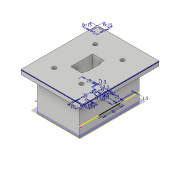
# Autodesk Inventor part: Chamber_coverslip_windowed.v8
Saved by Autodesk Inventor 2017 (Build 210142000, 142)
## iProperties
Created: 2016-07-27
Part Number: Chamber_coverslip_windowed.v8
Material: Generic
Document SubType Name: Modeling
Designer: Craggles
Density: 1 g/cm^3
Appearance: Default
Author: Craggles
Autodesk Inventor part; units mm, degrees
ref_plane "Work Plane1" through (0, 0, 0) normal (0, 0, 1) x (1, 0, 0)
sketch "Sketch1" plane through (0, 0, 0) normal (0, 0, 1) x (1, 0, 0)
  line L0 (45.9471, 19.6712) -> (70.9471, 19.6712)
  line L1 (70.9471, 19.6712) -> (70.9471, 19.8412)
  line L2 (70.9471, 19.8412) -> (45.9471, 19.8412)
  line L3 (45.9471, 19.8412) -> (45.9471, 19.6712)
  line L4 (45.9471, 19.8412) -> (45.9471, 23.669)
  line L5 (45.9471, 23.669) -> (23.5373, 23.669)
  line L6 (24.9679, 22.7263) -> (18.8195, 16.5991) construction
  line L7 (24.9679, 22.7263) -> (19.9679, 22.7263) construction
  line L8 (23.5373, 23.669) -> (24.9679, 22.7263) construction
  line L9 (18.8195, 16.5991) -> (13.8195, 16.5991) construction
  line L10 (13.8195, 16.5991) -> (19.9679, 22.7263)
  line L11 (19.9679, 22.7263) -> (20.9138, 23.669)
  line L12 (20.9138, 23.669) -> (23.5373, 23.669)
  line L13 (63.0355, 15.6366) -> (64.3758, 14.2916) construction
  line L14 (45.9471, 19.6712) -> (43.098, 19.6712) construction
  line L15 (63.0355, 15.6366) -> (65.8803, 15.6366) construction
  line L16 (65.8803, 15.6366) -> (65.8803, 19.8412) construction
  line L17 (72.2599, 24.8293) -> (14.1174, 24.8293)
  line L18 (69.6308, 12.9562) -> (67.6555, 14.9641) construction
  line L19 (69.6308, 12.9562) -> (72.4756, 12.9562) construction
  line L20 (67.6555, 14.9641) -> (70.5003, 14.9641) construction
  line L21 (70.5003, 14.9641) -> (72.4756, 12.9562) construction
  line L22 (70.9471, 14.5099) -> (75.9471, 14.5099) construction
  line L23 (75.9471, 14.5099) -> (75.9471, 24.8293) construction
  line L24 (75.9471, 24.8293) -> (72.2599, 24.8293)
  line L25 (13.8195, 16.5991) -> (11.7231, 14.5099)
  line L26 (11.7231, 14.5099) -> (6.7231, 14.5099) construction
  line L27 (6.7231, 14.5099) -> (6.7231, 24.8293) construction
  line L28 (6.7231, 24.8293) -> (14.1174, 24.8293)
  line L29 (75.9471, 24.8293) -> (6.7231, 24.8293) construction
  line L30 (6.7231, 24.8293) -> (6.7231, 67.9116) construction
  line L31 (6.7231, 67.9116) -> (75.9471, 67.9116)
  line L32 (75.9471, 67.9116) -> (75.9471, 24.8293) construction
  line L33 (11.7231, 14.5099) -> (5.1021, 7.9116)
  line L34 (5.1021, 7.9116) -> (3.1021, 7.9116)
  line L35 (3.1021, 7.9116) -> (3.1021, 67.9116)
  line L36 (3.1021, 67.9116) -> (6.7231, 67.9116)
  line L37 (72.4756, 12.9562) -> (75.9471, 9.4274) construction
  line L38 (5.1021, 7.9116) -> (77.4383, 7.9116) construction
  line L39 (77.4383, 7.9116) -> (75.9471, 9.4274) construction
  line L40 (77.4383, 7.9116) -> (77.4383, 67.9116)
  line L41 (77.4383, 67.9116) -> (75.9471, 67.9116)
  line L42 (77.4383, 7.9116) -> (79.4383, 7.9116)
  line L43 (79.4383, 7.9116) -> (79.4383, 67.9116)
  line L44 (79.4383, 67.9116) -> (77.4383, 67.9116)
  line L45 (70.9471, 19.8412) -> (77.4383, 19.8139)
  line L46 (70.9471, 19.8412) -> (71.4471, 19.8412)
  line L47 (70.9471, 19.8412) -> (71.4471, 19.8412) construction
  line L48 (71.4471, 19.8412) -> (71.4471, 14.0016)
  line L49 (71.4471, 14.0016) -> (77.4383, 7.9116)
  line L50 (45.9471, 19.8412) -> (67.9471, 19.8412)
  line L51 (67.9471, 19.8412) -> (67.9471, 17.5594)
  line L52 (67.9471, 17.5594) -> (71.4471, 14.0016)
  point P0 (0, 0)
  dimension "d0" = 25
  dimension "d1" = 0.17
  dimension "d2" = 5
  dimension "d3" = 5
  dimension "d4" = 2.8492
  dimension "d5" = 2.8448
  dimension "d7" = 2.8448
  dimension "d8" = 2.8448
  dimension "d11" = 5
  dimension "d13" = 5
  dimension "d49" = 2
  dimension "d50" = 2
  dimension "d51" = 90
  dimension "d52" = 0.5
  dimension "d53" = 0
  dimension "d54" = 90
  dimension "d175" = 60
  dimension "d199" = 22
  constraints: 106 end point, 15 horizontal, 8 perpendicular, 8 point on line, 6 parallel, 4 collinear
  measures "d0" distance of L2.end L1.end
  measures "d1" distance of L1.end L0.end
  measures "d2" distance of L6.start L7.end
  measures "d3" distance of L6.end L9.end
  measures "d4" distance of L0.start L14.end
  measures "d5" distance of L13.start L15.end
  measures "d7" distance of L18.start L19.end
  measures "d8" distance of L18.end L20.end
  measures "d11" distance of L22.start L23.start
  measures "d13" distance of L25.end L26.end
  measures "d49" distance of L33.end L34.end
  measures "d50" distance of L38.end L42.end
  measures "d51" angle of L43 L42
  measures "d52" distance of L1.end L46.end
  measures "d53" distance between parallel lines of L46 L47
  measures "d54" angle of L46 L48
  measures "d175" distance between parallel lines of L36 L34
  measures "d199" distance of L2.end L50.end
extrude "Extrusion1" add sketch "Sketch1" along normal mid plane 59.125 contours L51 L2 L1 L0 | L0 L1 L45 L48 L52 L51 | L4 L5 L12 L11 L10 L25 L33 L34 L35 L36 L31 L41 L40 L45 L48 L46 L2 | L46 L48 L45 | L48 L45 L40 L49 | L40 L44 L43 L42
sketch "Sketch3" plane through (0, 0, -29.5625) normal (0, 0, -1) x (-1, 0, 0)
  line L0 (-79.4383, 7.9116) -> (-77.4383, 7.9116) projected
  line L1 (-3.1021, 67.9116) -> (-79.4383, 67.9116)
  line L2 (-79.4383, 67.9116) -> (-79.4383, 7.9116)
  line L3 (-79.4383, 7.9116) -> (-3.1021, 7.9116)
  line L4 (-3.1021, 7.9116) -> (-3.1021, 67.9116)
  point P0 (-3.1021, 7.9116)
  constraints: 8 end point, 2 parallel, 1 horizontal, 1 perpendicular
extrude "End" add sketch "Sketch3" along normal blind 25
sketch "Sketch4" plane through (0, 0, 29.5625) normal (0, 0, 1) x (1, 0, 0)
  line L0 (3.1021, 67.9116) -> (3.1021, 7.9116) projected
  line L1 (79.4383, 7.9116) -> (3.1021, 7.9116)
  line L2 (3.1021, 7.9116) -> (3.1021, 67.9116)
  line L3 (3.1021, 67.9116) -> (79.4383, 67.9116)
  line L4 (79.4383, 67.9116) -> (79.4383, 7.9116)
  constraints: 8 end point, 2 parallel, 1 horizontal, 1 perpendicular
extrude "EndII" add sketch "Sketch4" along normal blind 25
sketch "Sketch7" plane through (45.9471, 19.8412, 29.5625) normal (0, -1, 0) x (1, 0, 0)
  line L0 (0, -18.5625) -> (5, -18.5625)
  line L1 (5, -18.5625) -> (5, -40.5625)
  line L2 (5, -40.5625) -> (0, -40.5625)
  line L3 (0, -40.5625) -> (0, -18.5625)
  line L4 (0, -59.125) -> (0, 0) projected
  point P0 (-45.9471, -29.5625)
  point P1 (0, -29.5625)
  dimension "d24" = 5
  dimension "d25" = 22
  constraints: 8 end point, 2 midpoint, 2 parallel, 1 horizontal, 1 perpendicular
  measures "d24" distance of L1.end L2.end
  measures "d25" distance of L0.end L1.end
extrude "Extrusion4" cut sketch "Sketch7" against normal up to surface (3.8278 mm away)
sketch "Sketch8" plane through (0, 0, 0) normal (0, 0, 1) x (1, 0, 0)
  point P0 (0, 0)
sketch "Sketch9" plane through (45.9471, 19.8412, -29.5625) normal (0, -1, 0) x (1, 0, 0)
  line L0 (25, 59.125) -> (25, 0) projected
  line L1 (0, 40.5625) -> (25, 40.5625)
  line L2 (25, 40.5625) -> (25, 41.5625)
  line L3 (25, 41.5625) -> (0, 41.5625)
  line L4 (0, 41.5625) -> (0, 40.5625)
  line L5 (0, 18.5625) -> (25, 18.5625)
  line L6 (25, 18.5625) -> (25, 17.5625)
  line L7 (25, 17.5625) -> (0, 17.5625)
  line L8 (0, 17.5625) -> (0, 18.5625)
  line L9 (0, 0) -> (0, 18.5625) projected
  line L10 (25, 17.5625) -> (0, 17.5625)
  line L11 (0, 17.5625) -> (0, 18.0625)
  line L12 (0, 18.0625) -> (25, 18.0625)
  line L13 (25, 18.0625) -> (25, 17.5625)
  line L14 (25, 41.5625) -> (0, 41.5625)
  line L15 (0, 41.5625) -> (0, 41.0625)
  line L16 (0, 41.0625) -> (25, 41.0625)
  line L17 (25, 41.0625) -> (25, 41.5625)
  point P0 (-45.9471, 29.5625)
  dimension "d28" = 1
  dimension "d29" = 1
  constraints: 32 end point, 8 parallel, 4 horizontal, 4 perpendicular, 3 point on line, 1 midpoint
  measures "d28" distance of L2.end L1.end
  measures "d29" distance of L5.end L6.end
extrude "Extrusion8" add sketch "Sketch9" along normal blind 0.1 contours L0 L16 L4 L3 | L0 L7 L8 L12
ref_plane "Work Plane2" through (45.9471, 26.669, -11) normal (0, -1, 0) x (1, 0, 0)
sketch "Sketch12" plane through (45.9471, 26.669, -11) normal (0, -1, 0) x (1, 0, 0)
  point P0 (-45.9471, 11)
sketch "Sketch14" plane through (45.9471, 26.669, -11) normal (0, -1, 0) x (1, 0, 0)
  line L0 (-42.845, -43.5625) -> (-42.845, 65.5625) projected
  line L1 (33.4911, -43.5625) -> (33.4911, 65.5625) projected
  line L2 (33.4911, 30) -> (33.4911, -8)
  line L3 (-42.845, -8) -> (-42.845, 30)
  line L4 (-42.845, -43.5625) -> (-42.845, 65.5625) projected
  line L5 (-42.845, 30) -> (-17.845, 30)
  line L6 (-17.845, 30) -> (-17.845, -8)
  line L7 (-17.845, -8) -> (-42.845, -8)
  line L8 (-42.845, -8) -> (-42.845, 30)
  line L9 (33.4911, 30) -> (8.4911, 30)
  line L10 (8.4911, 30) -> (8.4911, -8)
  line L11 (8.4911, -8) -> (33.4911, -8)
  line L12 (33.4911, -8) -> (33.4911, 30)
  line L13 (-17.845, 30) -> (-17.845, -8)
  line L14 (8.4911, -8) -> (8.4911, 30)
  line L15 (-17.845, 30) -> (-15.845, 30)
  line L16 (-15.845, 30) -> (-15.845, -8)
  line L17 (-15.845, -8) -> (-17.845, -8)
  line L18 (-17.845, -8) -> (-17.845, 30)
  line L19 (8.4911, 30) -> (6.4911, 30)
  line L20 (6.4911, 30) -> (6.4911, -8)
  line L21 (6.4911, -8) -> (8.4911, -8)
  line L22 (8.4911, -8) -> (8.4911, 30)
  line L23 (-15.845, -8) -> (-15.845, 30)
  line L24 (6.4911, 30) -> (6.4911, -8)
  line L25 (-15.845, -8) -> (-15.845, 30)
  line L26 (-15.845, 30) -> (-15.845, -8)
  line L27 (0, 22) -> (0, 40.5625) projected
  line L28 (-17.845, -8) -> (0, -8)
  line L29 (0, -8) -> (0, 30)
  line L30 (0, 30) -> (-17.845, 30)
  line L31 (-17.845, 30) -> (-17.845, -8)
  line L32 (5, 22) -> (5, 0) projected
  line L33 (0, 22) -> (5, 22)
  line L34 (5, 22) -> (5, 0)
  line L35 (5, 0) -> (0, 0)
  line L36 (0, 0) -> (0, 22)
  line L37 (1.5, 31.5) -> (-17.345, 31.5)
  line L38 (-17.345, 31.5) -> (-17.345, -9.5)
  line L39 (-17.345, -9.5) -> (1.5, -9.5)
  line L40 (1.5, -9.5) -> (1.5, 31.5)
  line L41 (6.5, 23.5) -> (0, 23.5)
  line L42 (0, 23.5) -> (0, -1.5)
  line L43 (0, -1.5) -> (6.5, -1.5)
  line L44 (6.5, -1.5) -> (6.5, 23.5)
  point P0 (-45.9471, 11)
  point P1 (-45.845, 65.5625)
  point P2 (36.4911, 65.5625)
  point P3 (-42.845, 11)
  point P4 (-42.845, 11)
  dimension "d55" = 38
  dimension "d58" = 25
  dimension "d59" = 38
  dimension "d60" = 25
  dimension "d135" = 2
  dimension "d136" = 2
  dimension "d153" = 1.5
  dimension "d154" = 1.5
  dimension "d155" = 1.5
  dimension "d156" = 1.5
  dimension "d157" = 1.5
  dimension "d158" = 1.5
  dimension "d159" = 1.5
  constraints: 80 end point, 19 parallel, 8 horizontal, 8 perpendicular, 3 point on line, 1 coincident, 1 midpoint, 6 other
  measures "d55" distance of L2.start L2.end
  measures "d58" distance of L6.end L7.end
  measures "d59" distance of L5.end L6.end
  measures "d60" distance of L11.end L10.end
  measures "d135" distance of L16.end L17.end
  measures "d136" distance of L21.end L20.end
  measures "d153" distance between parallel lines of L38 L16
  measures "d154" distance between parallel lines of L39 L28
  measures "d155" distance between parallel lines of L40 L29
  measures "d156" distance between parallel lines of L37 L30
  measures "d157" distance between parallel lines of L33 L41
  measures "d158" distance between parallel lines of L32 L44
  measures "d159" distance between parallel lines of L43 L35
extrude "Extrusion10" cut sketch "Sketch14" against normal blind 5 contours L0 L5 L6 L7
ref_plane "Work Plane3" through (0.1021, 7.9116, 54.5625) normal (0, -1, 0) x (1, 0, 0)
sketch "Sketch17" plane through (3.1021, 67.9116, -54.5625) normal (0, 1, 0) x (1, 0, 0)
  line L0 (82.3362, -109.125) -> (0, -109.125) projected
  line L1 (0, -109.125) -> (76.3362, -109.125)
  line L2 (76.3362, -109.125) -> (76.3362, 0)
  line L3 (76.3362, 0) -> (0, 0)
  line L4 (0, 0) -> (0, -109.125)
  point P0 (-3.1021, -54.5625)
  constraints: 8 end point, 2 parallel, 1 horizontal, 1 perpendicular
extrude "Extrusion11" add sketch "Sketch17" along normal blind 10
ref_plane "Work Plane4" through (3.1021, 77.9116, -54.5625) normal (0, 1, 0) x (1, 0, 0)
sketch "Sketch18" plane through (3.1021, 77.9116, -54.5625) normal (0, 1, 0) x (1, 0, 0)
  line L0 (0, 0) -> (-15, 0) construction
  line L1 (-15, 0) -> (-15, 15)
  line L2 (-15, 15) -> (0, 15)
  line L3 (0, 15) -> (0, 0) construction
  line L4 (82.3362, -109.125) -> (97.3362, -109.125) construction
  line L5 (97.3362, -109.125) -> (97.3362, -124.125)
  line L6 (97.3362, -124.125) -> (82.3362, -124.125)
  line L7 (82.3362, -124.125) -> (82.3362, -109.125) construction
  line L8 (97.3362, -124.125) -> (-15, -124.125)
  line L9 (-15, -124.125) -> (-15, 15)
  line L10 (-15, 15) -> (97.3362, 15)
  line L11 (97.3362, 15) -> (97.3362, -124.125)
  line L12 (-15, 15) -> (-13, 15)
  line L13 (-13, 15) -> (-13, 13)
  line L14 (-13, 13) -> (-15, 13)
  line L15 (-15, 13) -> (-15, 15)
  line L16 (97.3362, -124.125) -> (95.3362, -124.125)
  line L17 (95.3362, -124.125) -> (95.3362, -122.125)
  line L18 (95.3362, -122.125) -> (97.3362, -122.125)
  line L19 (97.3362, -122.125) -> (97.3362, -124.125)
  line L20 (-13, 13) -> (95.3362, 13)
  line L21 (95.3362, 13) -> (95.3362, -122.125)
  line L22 (95.3362, -122.125) -> (-13, -122.125)
  line L23 (-13, -122.125) -> (-13, 13)
  line L24 (-13, 15) -> (-15, 15)
  line L25 (-15, 15) -> (-15, -124.125)
  line L26 (-15, -124.125) -> (-13, -124.125)
  line L27 (-13, -124.125) -> (-13, 15)
  line L28 (97.3362, 15) -> (95.3362, 15)
  line L29 (95.3362, 15) -> (95.3362, -124.125)
  line L30 (95.3362, -124.125) -> (97.3362, -124.125)
  line L31 (97.3362, -124.125) -> (97.3362, 15)
  point P0 (-3.1021, -54.5625)
  point P1 (0, 0)
  dimension "d106" = 15
  dimension "d107" = 15
  dimension "d108" = 15
  dimension "d109" = 15
  dimension "d110" = 2
  dimension "d111" = 2
  dimension "d112" = 2
  dimension "d113" = 2
  constraints: 64 end point, 16 parallel, 8 horizontal, 8 perpendicular, 1 coincident
  measures "d106" distance of L1.end L2.end
  measures "d107" distance of L0.end L1.end
  measures "d108" distance of L5.end L6.end
  measures "d109" distance of L4.end L5.end
  measures "d110" distance of L13.end L14.end
  measures "d111" distance of L12.end L13.end
  measures "d112" distance of L17.end L18.end
  measures "d113" distance of L16.end L17.end
extrude "Extrusion15" add sketch "Sketch18" along normal blind 1
extrude "Extrusion16" add sketch "Sketch18" against normal blind 7.5 contours L1 L14 L23 L27 L8 L9 | L1 L2 L13 L14 | L13 L2 L10 L29 L20 | L27 L22 L17 L6 L8 | L29 L10 L11 L5 L18 L21 | L18 L5 L6 L17
extrude "Extrusion17" cut sketch "Sketch14" along normal blind 5 contours L10 L9 L1 L11
sketch "Sketch15" plane through (3.1021, 7.9116, -54.5625) normal (0, -1, 0) x (1, 0, 0)
  line L0 (63.1681, 17.0625) -> (38.1681, 17.0625)
  line L1 (38.1681, 17.0625) -> (38.1681, 42.0625)
  line L2 (38.1681, 42.0625) -> (63.1681, 42.0625)
  line L3 (63.1681, 42.0625) -> (63.1681, 17.0625)
  line L4 (38.1681, 42.0625) -> (13.1681, 42.0625)
  line L5 (13.1681, 42.0625) -> (13.1681, 67.0625)
  line L6 (13.1681, 67.0625) -> (38.1681, 67.0625)
  line L7 (38.1681, 67.0625) -> (38.1681, 42.0625)
  line L8 (38.1681, 17.0625) -> (13.1681, 17.0625)
  line L9 (13.1681, 17.0625) -> (13.1681, 42.0625)
  line L10 (13.1681, 42.0625) -> (38.1681, 42.0625)
  line L11 (38.1681, 42.0625) -> (38.1681, 17.0625)
  line L12 (38.1681, 67.0625) -> (13.1681, 67.0625)
  line L13 (13.1681, 67.0625) -> (13.1681, 92.0625)
  line L14 (13.1681, 92.0625) -> (38.1681, 92.0625)
  line L15 (38.1681, 92.0625) -> (38.1681, 67.0625)
  line L16 (63.1681, 42.0625) -> (38.1681, 42.0625)
  line L17 (38.1681, 42.0625) -> (38.1681, 67.0625)
  line L18 (38.1681, 67.0625) -> (63.1681, 67.0625)
  line L19 (63.1681, 67.0625) -> (63.1681, 42.0625)
  line L20 (63.1681, 67.0625) -> (38.1681, 67.0625)
  line L21 (38.1681, 67.0625) -> (38.1681, 92.0625)
  line L22 (38.1681, 92.0625) -> (63.1681, 92.0625)
  line L23 (63.1681, 92.0625) -> (63.1681, 67.0625)
  line L24 (63.1681, 92.0625) -> (38.1681, 92.0625)
  line L25 (38.1681, 92.0625) -> (13.1681, 92.0625)
  line L26 (76.3362, 0) -> (0, 0) projected
  line L27 (57.3362, 73.5625) -> (57.3362, 35.5625) projected
  point P0 (69.44, 116.6702)
  point P1 (19.44, 116.6702)
  point P2 (38.1681, 0)
  point P3 (63.1681, 54.5625)
  point P4 (57.3362, 54.5625)
  dimension "d80" = 25
  dimension "d81" = 25
  dimension "d82" = 25
  dimension "d83" = 25
  dimension "d84" = 25
  dimension "d85" = 25
  dimension "d86" = 25
  dimension "d87" = 25
  dimension "d88" = 25
  dimension "d89" = 25
  dimension "d90" = 25
  dimension "d91" = 25
  constraints: 52 end point, 12 parallel, 8 horizontal, 6 perpendicular, 3 midpoint, 1 horizontal alignment, 1 vertical alignment
  measures "d80" distance of L1.end L2.end
  measures "d81" distance of L0.end L1.end
  measures "d82" distance of L5.end L6.end
  measures "d83" distance of L4.end L5.end
  measures "d84" distance of L9.end L10.end
  measures "d85" distance of L8.end L9.end
  measures "d86" distance of L13.end L14.end
  measures "d87" distance of L12.end L13.end
  measures "d88" distance of L12.start L18.end
  measures "d89" distance of L16.end L12.start
  measures "d90" distance of L21.end L22.end
  measures "d91" distance of L20.end L21.end
hole "Hole2" at (66.2702, 7.9116, -37.5) at (16.2702, 7.9116, -37.5) at (66.2702, 7.9116, 37.5) at (16.2702, 7.9116, 37.5) direction (0, 1, 0) diameter 7 end through all counterbore diameter 11.5 counterbore depth 40
sketch "Sketch19" plane through (3.1021, 7.9116, -54.5625) normal (0, -1, 0) x (1, 0, 0)
  line L0 (64.845, 25) -> (42.845, 25) projected
  line L1 (53.845, 25) -> (18.845, 25)
  line L2 (18.845, 25) -> (18.845, 22)
  line L3 (18.845, 22) -> (53.845, 22)
  line L4 (53.845, 22) -> (53.845, 25)
  line L5 (76.3362, 0) -> (0, 0) projected
  line L6 (19.845, 0) -> (52.845, 0)
  line L7 (52.845, 0) -> (52.845, 22)
  line L8 (52.845, 22) -> (19.845, 22)
  line L9 (19.845, 22) -> (19.845, 0)
  line L10 (52.845, 0) -> (54.345, 0)
  line L11 (54.345, 0) -> (54.345, 22)
  line L12 (54.345, 22) -> (52.845, 22)
  line L13 (52.845, 22) -> (52.845, 0)
  line L14 (19.845, 0) -> (18.345, 0)
  line L15 (18.345, 0) -> (18.345, 22)
  line L16 (18.345, 22) -> (19.845, 22)
  line L17 (19.845, 22) -> (19.845, 0)
  point P0 (-3.1021, 54.5625)
  point P1 (67.845, 25)
  point P2 (36.345, 22)
  dimension "d126" = 35
  dimension "d127" = 3
  dimension "d128" = 33
  dimension "d139" = 1.5
  dimension "d140" = 1.5
  constraints: 32 end point, 8 parallel, 4 horizontal, 4 perpendicular, 3 midpoint, 3 point on line
  measures "d126" distance of L3.end L2.end
  measures "d127" distance of L2.end L1.end
  measures "d128" distance of L8.end L7.end
  measures "d139" distance of L12.end L11.end
  measures "d140" distance of L15.end L16.end
extrude "Extrusion18" cut sketch "Sketch19" against normal blind 16.5 contours L4 L3 L2 L1 L0
extrude "Extrusion19" cut sketch "Sketch14" along normal blind 3.1375 and the other way blind 27.9705 contours L16 L30 L27 L29 L28 | L29 L33 L40 L35 | L40 L33 L32 L35
extrude "Extrusion20" cut sketch "Sketch19" against normal up to surface (15.7574 mm away) contours L7 L5 L9 L3
extrude "Extrusion21" cut sketch "Sketch19" against normal blind 1.5 contours L12 L11 L5 L7 L3 | L3 L9 L5 L15 L16
sketch "Sketch23" plane through (3.1021, 78.9116, -54.5625) normal (0, 1, 0) x (1, 0, 0)
  line L0 (26, -34.5625) -> (46.845, -34.5625)
  line L1 (46.845, -34.5625) -> (46.845, -74.5625)
  line L2 (46.845, -74.5625) -> (26, -74.5625)
  line L3 (26, -74.5625) -> (26, -34.5625)
  line L4 (27, -73.5625) -> (27, -35.5625) projected
  line L5 (45.845, -73.5625) -> (27, -73.5625) projected
  line L6 (45.845, -35.5625) -> (45.845, -43.5625) projected
  line L7 (27, -35.5625) -> (45.845, -35.5625) projected
  line L8 (48.845, -66.5625) -> (44.845, -66.5625)
  line L9 (44.845, -66.5625) -> (44.845, -42.5625)
  line L10 (44.845, -42.5625) -> (48.845, -42.5625)
  line L11 (48.845, -42.5625) -> (48.845, -66.5625)
  line L12 (47.845, -65.5625) -> (47.845, -43.5625) projected
  line L13 (45.845, -43.5625) -> (47.845, -43.5625) projected
  line L14 (47.845, -65.5625) -> (45.845, -65.5625) projected
  point P0 (-3.1021, -54.5625)
  dimension "d143" = 1
  dimension "d144" = 1
  dimension "d145" = 1
  dimension "d146" = 1
  dimension "d147" = 1
  dimension "d148" = 1
  dimension "d149" = 1
  dimension "d150" = 1
  constraints: 16 end point, 4 parallel, 2 horizontal, 2 perpendicular
  measures "d143" distance between parallel lines of L4 L3
  measures "d144" distance between parallel lines of L2 L5
  measures "d145" distance between parallel lines of L6 L1
  measures "d146" distance between parallel lines of L7 L0
  measures "d147" distance between parallel lines of L6 L9
  measures "d148" distance between parallel lines of L12 L11
  measures "d149" distance between parallel lines of L13 L10
  measures "d150" distance between parallel lines of L8 L14
extrude "Extrusion22" cut sketch "Sketch23" against normal blind 28
extrude "Extrusion23" cut sketch "Sketch14" against normal blind 3 and the other way blind 6 contours L38 L15 L16 L17 | L17 L28 L29 L43 L40 L39 L38 | L38 L37 L27 L30 L15 | L16 L30 L27 L29 L28 | L27 L37 L40 L41 | L29 L35 L40 L43 | L40 L35 L32 L33 L41 L20 L43 | L41 L40 L33 L27 | L20 L41 L44 L43
fillet "Fillet1" radius 1.44 7 edges at (47.4471, 20.669, 16.5) (49.9471, 20.669, 12.5) (52.4471, 20.669, 0) (49.9471, 20.669, -12.5) (47.4471, 20.669, -16.5) (46.6971, 20.669, -20.5) (46.6971, 20.669, 20.5) curvature continuous yes
sketch "Sketch25" plane through (28.6021, 29.669, -20.5) normal (0, 0, 1) x (1, 0, 0)
  point P0 (-28.6021, -29.669)
sketch "Sketch26" plane through (30.1021, 54.6395, -19) normal (0, 0, 1) x (1, 0, 0)
  line L0 (15.845, -30.9705) -> (-8.155, -30.9705) projected
  line L1 (17.345, -24.9705) -> (-1.5, -24.9705) projected
  line L2 (15.845, -30.9705) -> (-1.5, -30.9705)
  line L3 (-1.5, -30.9705) -> (-1.5, -24.9705)
  line L4 (-1.5, -24.9705) -> (15.845, -24.9705)
  line L5 (15.845, -24.9705) -> (15.845, -30.9705)
  line L6 (-1.5, -24.9705) -> (15.845, -24.9705)
  line L7 (15.845, -24.9705) -> (15.845, -27.9705)
  line L8 (15.845, -27.9705) -> (-1.5, -27.9705)
  line L9 (-1.5, -27.9705) -> (-1.5, -24.9705)
  line L10 (-40, 23.2721) -> (68.3362, 23.2721) projected
  line L11 (15.845, -24.9705) -> (-2.9952, -24.9705)
  line L12 (-2.9952, -24.9705) -> (-2.9952, 23.2721)
  line L13 (-2.9952, 23.2721) -> (15.845, 23.2721)
  line L14 (15.845, 23.2721) -> (15.845, -24.9705)
  line L15 (15.845, -24.9705) -> (-2.9952, -24.9705)
  line L16 (-2.9952, -24.9705) -> (-2.9952, -0.8492)
  line L17 (-2.9952, -0.8492) -> (15.845, -0.8492)
  line L18 (15.845, -0.8492) -> (15.845, -24.9705)
  line L19 (-2.9952, -0.8492) -> (15.845, -0.8492)
  line L20 (15.845, -0.8492) -> (15.845, 23.2721)
  line L21 (15.845, 23.2721) -> (-2.9952, 23.2721)
  line L22 (-2.9952, 23.2721) -> (-2.9952, -0.8492)
  line L23 (0, 0) -> (0, -24.9705) projected
  line L24 (15.845, -24.9705) -> (15.845, 0) projected
  line L25 (0, 0) -> (15.845, 0)
  line L26 (15.845, 0) -> (15.845, -5)
  line L27 (15.845, -5) -> (0, -5)
  line L28 (0, -5) -> (0, 0)
  point P0 (-30.1021, -54.6395)
  dimension "d171" = 5
  constraints: 48 end point, 12 parallel, 6 horizontal, 6 perpendicular, 2 midpoint, 2 point on line
  measures "d171" distance of L25.end L26.end
extrude "Extrusion25" cut sketch "Sketch26" against normal blind 39.2125 contours L27 L23 L17 L14 | L17 L23 L25 L14
sketch "Sketch28" plane through (30.1021, 54.6395, -19) normal (0, 0, 1) x (1, 0, 0)
  point P0 (-30.1021, -54.6395)
sketch "Sketch29" plane through (30.1021, 54.6395, -19) normal (0, 0, 1) x (1, 0, 0)
  line L0 (15.845, 0) -> (0, 0) projected
  line L1 (7.9225, 0) -> (-2.0775, 0)
  line L2 (-2.0775, 0) -> (-2.0775, -10)
  line L3 (-2.0775, -10) -> (7.9225, -10)
  line L4 (7.9225, -10) -> (7.9225, 0)
  line L5 (7.9225, 0) -> (22.3455, 0)
  line L6 (22.3455, 0) -> (22.3455, -10)
  line L7 (22.3455, -10) -> (7.9225, -10)
  line L8 (7.9225, -10) -> (7.9225, 0)
  point P0 (-30.1021, -54.6395)
  dimension "d177" = 10
  dimension "d178" = 10
  dimension "d179" = 14.423
  constraints: 16 end point, 4 parallel, 2 horizontal, 2 perpendicular, 1 midpoint, 1 point on line
  measures "d177" distance of L3.end L2.end
  measures "d178" distance of L2.end L1.end
  measures "d179" distance of L6.end L7.end
extrude "Extrusion27" cut sketch "Sketch29" against normal up to surface (73.5625 mm away) from surface at 38
sketch "Sketch30" plane through (45.9471, 54.6395, -11) normal (0, -1, 0) x (1, 0, 0)
  point P0 (-45.9471, 11)
sketch "Sketch31" plane through (45.9471, 54.6395, -11) normal (0, -1, 0) x (1, 0, 0)
  line L0 (-15.845, 30) -> (0, 30) projected
  line L1 (-15.845, 30) -> (12.155, 30)
  line L2 (12.155, 30) -> (12.155, -8)
  line L3 (12.155, -8) -> (-15.845, -8)
  line L4 (-15.845, -8) -> (-15.845, 30)
  line L5 (0, -8) -> (-15.845, -8) projected
  line L6 (5, 22) -> (5, 0) projected
  point P0 (-45.9471, 11)
  dimension "d188" = 28
  constraints: 8 end point, 1 collinear, 1 horizontal, 1 parallel, 1 perpendicular
  measures "d188" distance between parallel lines of L4 L2
extrude "Extrusion28" cut sketch "Sketch31" along normal blind 23.3375
sketch "Sketch32" plane through (30.1021, 54.6395, -19) normal (0, 0, 1) x (1, 0, 0)
  line L0 (28, -24.9705) -> (0, -24.9705)
  line L1 (0, -24.9705) -> (0, 0)
  line L2 (0, 0) -> (28, 0)
  line L3 (28, 0) -> (28, -24.9705)
  line L4 (28, 0) -> (0, 0) projected
  line L5 (0, -24.9705) -> (0, -10) projected
  line L6 (28, 0) -> (28, -23.3375) projected
  line L7 (17.345, -24.9705) -> (-1.5, -24.9705) projected
  line L8 (28, 0) -> (0, 0)
  line L9 (0, 0) -> (0, -23.9705)
  line L10 (0, -23.9705) -> (28, -23.9705)
  line L11 (28, -23.9705) -> (28, 0)
  point P0 (-30.1021, -54.6395)
  point P1 (28, -22.3375)
  dimension "d193" = 1
  constraints: 16 end point, 4 collinear, 4 parallel, 2 horizontal, 2 perpendicular, 1 point on line
  measures "d193" distance between parallel lines of L0 L10
extrude "Extrusion29" [suppressed]
chamfer "Chamfer1" distance 6.7625 angle 45 3 edges at (52.0246, 31.302, 19) (58.1021, 31.302, 0) (52.0246, 31.302, -19)
fillet "Fillet5" [suppressed]
sketch "Sketch33" plane through (45.9471, 19.8412, 11) normal (0, -1, 0) x (1, 0, 0)
  line L0 (0, 0.5) -> (22, 0.5) projected
  line L1 (25.5, -40.5625) -> (25.5, 18.5625) projected
  line L2 (0, 0.5) -> (25.5, 0.5)
  line L3 (25.5, 0.5) -> (25.5, -22.4897)
  line L4 (25.5, -22.4897) -> (0, -22.4897)
  line L5 (0, -22.4897) -> (0, 0.5)
  point P0 (-45.9471, -11)
  point P1 (25, 0.5)
  constraints: 8 end point, 2 parallel, 1 horizontal, 1 perpendicular, 1 point on line
extrude "Extrusion30" [suppressed]
ref_plane "Work Plane6" through (5.1021, 12.9116, 29.5625) normal (0, -1, 0) x (1, 0, 0)
sketch "Sketch34" plane through (5.1021, 12.9116, 29.5625) normal (0, -1, 0) x (1, 0, 0)
  line L0 (74.3362, -84.125) -> (74.3362, 25) projected
  line L1 (74.3362, 25) -> (-8.1021, 25)
  line L2 (-8.1021, 25) -> (-8.1021, -84.125)
  line L3 (-8.1021, -84.125) -> (74.3362, -84.125)
  line L4 (74.3362, -84.125) -> (74.3362, 25)
  point P0 (-5.1021, -29.5625)
  constraints: 8 end point, 2 parallel, 1 horizontal, 1 perpendicular
extrude "Extrusion31" [suppressed]
equation "\"d106\" = d109"
equation "\"d107\" = d108"
body "Solid1"
